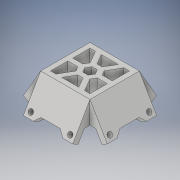
# Autodesk Inventor part: 4-Tool_Upper
Saved by Autodesk Inventor 2019 (Build 230136000, 136)
## iProperties
Created: 2021-01-31
Part Number: 4-Tool_Upper
Material: Generic
Document SubType Name: Modeling
Designer: zhanb
Density: 1 g/cm^3
Appearance: Default
Author: zhanb
Autodesk Inventor part; units mm, degrees
ref_plane "YZ Plane" through (0, 0, 0) normal (1, 0, 0) x (0, 1, 0)
ref_plane "XZ Plane" through (0, 0, 0) normal (0, 1, 0) x (-1, 0, 0)
ref_plane "XY Plane" through (0, 0, 0) normal (0, 0, 1) x (1, 0, 0)
sketch "Sketch2" plane through (0, 0, 0) normal (1, 0, 0) x (0, 1, 0)
  line L0 (-38.1, 25.4) -> (38.1, 25.4) construction
  line L1 (38.1, 25.4) -> (38.1, -25.4) construction
  line L2 (38.1, -25.4) -> (-38.1, -25.4) construction
  line L3 (-38.1, -25.4) -> (-38.1, 25.4) construction
  line L4 (-38.1, 25.4) -> (38.1, -25.4) construction
  line L5 (38.1, 25.4) -> (-38.1, -25.4) construction
  line L6 (38.1, 25.4) -> (-60.8867, 82.55) construction
  line L7 (-60.8867, 82.55) -> (-67.2367, 71.5515) construction
  line L8 (-67.2367, 71.5515) -> (15.1277, 23.9984) construction
  line L9 (38.1, 0) -> (82.0941, 0) construction
  line L10 (82.0941, 0) -> (38.1, 25.4) construction
  line L11 (38.1, 25.4) -> (7.3041, 43.18)
  line L12 (7.3041, 43.18) -> (4.1291, 37.6807)
  line L13 (0.9541, 32.1815) -> (0.9541, 0) construction
  line L14 (0.9541, 0) -> (15.1277, 0) construction
  line L15 (38.1, 25.4) -> (38.1, 0)
  line L16 (0.9541, 32.1815) -> (15.1277, 23.9984) construction
  line L17 (15.1277, 23.9984) -> (15.1277, 0)
  line L18 (15.1277, 0) -> (38.1, 0)
  line L19 (4.1291, 37.6807) -> (15.1277, 31.3307)
  line L20 (15.1277, 31.3307) -> (15.1277, 23.9984)
  line L21 (4.1291, 37.6807) -> (0.9541, 32.1815) construction
  point P0 (0, 0)
  dimension "d2" = 76.2
  dimension "d3" = 50.8
  dimension "d4" = 12.7
  dimension "d5" = 30
  dimension "d6" = 114.3
  dimension "d7" = 35.56
  dimension "d32" = 6.35
  dimension "d33" = 12.7
  constraints: 44 end point, 11 perpendicular, 3 collinear, 3 midpoint, 3 parallel, 2 horizontal, 2 point on line
  measures "d2" distance of L1.end L2.end
  measures "d3" distance of L0.end L1.end
  measures "d4" distance of L6.end L7.end
  measures "d5" angle of L9 L10
  measures "d6" distance of L0.end L6.end
  measures "d7" distance of L0.end L11.end
  measures "d32" distance between parallel lines of L11 L19
  measures "d33" distance of L19.end L12.end
extrude "Extrusion1" add sketch "Sketch2" along normal mid plane 50.8
pattern_circular "Circular Pattern1" count 4 over 360 about axis through (0, -10, 0) along (0, 1, 0) of "Extrusion1"
sketch "Sketch5" plane through (-25.4, 38.1, -25.4) normal (-0.8660254, 0.5, 0) x (0, 0, 1)
  circle A0 centre (5.08, -30.48) radius 2.5527
  circle A1 centre (45.72, -30.48) radius 2.5527
  line L0 (5.08, -30.48) -> (45.72, -30.48) construction
  line L1 (50.8, 0) -> (0, 0) construction
  point P0 (25.4, -30.48)
  point P1 (25.4, 0)
  dimension "d20" = 40.64
  dimension "d21" = 5.1054
  dimension "d22" = 5.1054
  dimension "d24" = 30.48
  constraints: 2 centre point, 2 coincident, 2 end point, 2 midpoint, 1 horizontal, 1 horizontal alignment, 1 vertical alignment
  measures "d20" distance of point (45.72, -30.48) point (5.08, -30.48)
  measures "d21" diameter of A0
  measures "d22" diameter of A1
  measures "d24" distance from line of L1 point (25.4, -30.48)
hole "Hole1" at (-40.64, 11.7035, -20.32) at (-40.64, 11.7035, 20.32) direction (0.8660254, -0.5, 0) diameter 5.1562 end through all
sketch "Sketch6" plane through (0, 0, 0) normal (0, 0, 1) x (1, 0, 0)
  line L0 (-34.9969, 8.7777) -> (-24.8369, 8.7777)
  line L1 (-24.8369, 8.7777) -> (-21.1707, 15.1277)
  line L2 (25.4, 15.1277) -> (-25.4, 15.1277) construction
  line L3 (-31.3307, 15.1277) -> (-34.9969, 8.7777)
  line L4 (-37.6807, 4.1291) -> (-31.3307, 15.1277) construction
  line L5 (-31.3307, 15.1277) -> (-21.1707, 15.1277)
  point P0 (0, 0)
  dimension "d34" = 6.35
  dimension "d35" = 10.16
  constraints: 8 end point, 2 collinear, 1 horizontal, 1 parallel, 1 point on line
  measures "d34" distance between parallel lines of L5 L0
  measures "d35" distance of L3.start L1.end
extrude "Extrusion3" add sketch "Sketch6" along normal mid plane 5.08
sketch "Sketch7" plane through (-43.18, 7.3041, -25.4) normal (-0.8660254, 0.5, 0) x (0, 0, 1)
  line L0 (22.86, 5.3677) -> (27.94, 5.3677) construction
  line L1 (10.16, 0) -> (15.5277, 5.3677)
  line L2 (15.5277, 5.3677) -> (35.2723, 5.3677)
  line L3 (35.2723, 5.3677) -> (40.64, 0)
  line L4 (40.64, 0) -> (10.16, 0)
  line L5 (0, 0) -> (50.8, 0) construction
  point P0 (25.4, 15.2644)
  point P1 (25.4, 5.3677)
  point P2 (25.4, 0)
  dimension "d38" = 45
  dimension "d39" = 10.16
  constraints: 8 end point, 4 midpoint, 3 collinear, 1 horizontal
  measures "d38" angle of L4 L1
  measures "d39" distance of L5.start L1.start
extrude "Extrusion4" cut sketch "Sketch7" against normal through all
sketch "Sketch8" plane through (-25.4, 38.1, 25.4) normal (0, 1, 0) x (1, 0, 0)
  line L0 (28.1496, 20.6375) -> (22.6504, 20.6375)
  line L1 (22.6504, 20.6375) -> (19.9007, 25.4)
  line L2 (19.9007, 25.4) -> (22.6504, 30.1625)
  line L3 (22.6504, 30.1625) -> (28.1496, 30.1625)
  line L4 (28.1496, 30.1625) -> (30.8993, 25.4)
  line L5 (30.8993, 25.4) -> (28.1496, 20.6375)
  line L6 (45.72, 45.72) -> (5.08, 45.72) construction
  line L7 (5.08, 45.72) -> (5.08, 5.08) construction
  line L8 (5.08, 5.08) -> (45.72, 5.08) construction
  line L9 (45.72, 5.08) -> (45.72, 45.72) construction
  line L10 (45.72, 45.72) -> (5.08, 5.08) construction
  line L11 (5.08, 45.72) -> (45.72, 5.08) construction
  line L12 (35.2987, 22.86) -> (45.72, 22.86)
  line L13 (45.72, 22.86) -> (45.72, 5.08)
  line L14 (45.72, 5.08) -> (40.0647, 5.08)
  line L15 (40.0647, 5.08) -> (32.549, 18.0975)
  line L16 (32.549, 18.0975) -> (35.2987, 22.86)
  line L17 (28.1496, 15.5575) -> (22.6504, 15.5575)
  line L18 (22.6504, 15.5575) -> (16.6012, 5.08)
  line L19 (34.1988, 5.08) -> (28.1496, 15.5575)
  line L20 (28.1496, 20.6375) -> (37.1318, 5.08) construction
  line L21 (10.7353, 5.08) -> (18.251, 18.0975)
  line L22 (18.251, 18.0975) -> (15.5013, 22.86)
  line L23 (15.5013, 22.86) -> (5.08, 22.86)
  line L24 (5.08, 22.86) -> (5.08, 5.08)
  line L25 (10.7353, 5.08) -> (5.08, 5.08)
  line L26 (45.72, 27.94) -> (35.2987, 27.94)
  line L27 (35.2987, 27.94) -> (32.549, 32.7025)
  line L28 (32.549, 32.7025) -> (40.0647, 45.72)
  line L29 (40.0647, 45.72) -> (45.72, 45.72)
  line L30 (45.72, 27.94) -> (45.72, 45.72)
  line L31 (30.8993, 25.4) -> (45.72, 25.4) construction
  line L32 (31.0826, 15.5575) -> (19.7174, 15.5575) construction
  line L33 (19.7174, 15.5575) -> (14.0349, 25.4) construction
  line L34 (14.0349, 25.4) -> (19.7174, 35.2425) construction
  line L35 (19.7174, 35.2425) -> (31.0826, 35.2425) construction
  line L36 (31.0826, 35.2425) -> (36.7651, 25.4) construction
  line L37 (36.7651, 25.4) -> (31.0826, 15.5575) construction
  line L38 (14.0349, 25.4) -> (5.08, 25.4) construction
  line L39 (25.4, 5.08) -> (25.4, 25.4) construction
  line L40 (28.1496, 35.2425) -> (34.1988, 45.72)
  line L41 (16.6012, 45.72) -> (22.6504, 35.2425)
  line L42 (28.1496, 35.2425) -> (22.6504, 35.2425)
  line L43 (15.5013, 27.94) -> (5.08, 27.94)
  line L44 (5.08, 27.94) -> (5.08, 45.72)
  line L45 (5.08, 45.72) -> (10.7353, 45.72)
  line L46 (10.7353, 45.72) -> (18.251, 32.7025)
  line L47 (15.5013, 27.94) -> (18.251, 32.7025)
  line L48 (31.0826, 35.2425) -> (37.1318, 45.72) construction
  line L49 (30.441, 11.5887) -> (34.8404, 14.1287) construction
  line L50 (34.1988, 5.08) -> (16.6012, 5.08)
  line L51 (34.1988, 45.72) -> (16.6012, 45.72)
  point P0 (25.4, 15.5575)
  point P1 (25.4, 20.6375)
  point P2 (32.6407, 12.8587)
  dimension "d42" = 9.525
  dimension "d46" = 40.64
  dimension "d47" = 40.64
  dimension "d48" = 5.08
  dimension "d49" = 5.08
  dimension "d50" = 5.08
  constraints: 104 end point, 12 point on line, 11 equal length, 10 horizontal, 9 midpoint, 9 perpendicular, 8 parallel, 7 collinear, 2 coincident, 1 vertical, 1 vertical alignment, 31 other
  measures "d42" distance between parallel lines of L3 L0
  measures "d46" distance of L6.end L7.end
  measures "d47" distance of L7.end L8.end
  measures "d48" distance of L49.start L49.end
  measures "d49" distance between parallel lines of L26 L12
  measures "d50" distance between parallel lines of L5 L16
extrude "Extrusion5" cut sketch "Sketch8" against normal through all
pattern_circular "Circular Pattern2" count 4 over 360 about axis through (0, -10, 0) along (0, 1, 0) of "Extrusion3", "Hole1", "Extrusion4"
equation "\"d47\" = d46"
equation "\"d49\" = d48"
equation "\"d50\" = d48"
body "Solid1"
